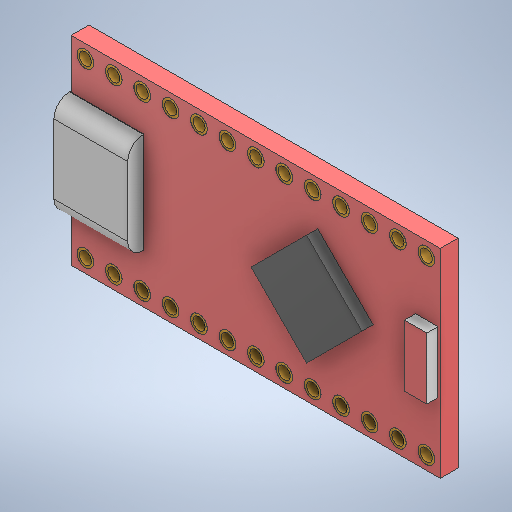
# Autodesk Inventor part: nrf52840
Saved by Autodesk Inventor 2025.2 (Build 292293000, 293)
## iProperties
Created: 2025-04-17
Part Number: nrf52840
Material: Generic
Document SubType Name: Modeling
Designer: Andreas
Density: 1 g/cm^3
Appearance: Default
Author: Andreas
Autodesk Inventor part; units mm, degrees
ref_plane "YZ Plane" through (0, 0, 0) normal (1, 0, 0) x (0, 1, 0)
ref_plane "XZ Plane" through (0, 0, 0) normal (0, 1, 0) x (-1, 0, 0)
ref_plane "XY Plane" through (0, 0, 0) normal (0, 0, 1) x (1, 0, 0)
sketch "Block1" plane through (0, 0, 0) normal (0, 0, 1) x (1, 0, 0)
  line L0 (0.0387, 6.6847) -> (0.0387, 12.8847)
  line L1 (0.2387, 6.6847) -> (0.2387, 12.8847)
  line L2 (1.1887, 12.9847) -> (1.1887, 6.5847)
  line L3 (1.8887, 6.5847) -> (1.8887, 12.9847)
  line L4 (2.8387, 12.8847) -> (2.8387, 6.6847)
  line L5 (3.0387, 12.8847) -> (3.0387, 6.6847)
  arc A0 (1.1887, 6.5847) -> (1.4887, 6.2847) centre (1.4887, 6.5847) ccw
  line L6 (1.4887, 6.2847) -> (1.5887, 6.2847)
  arc A1 (1.5887, 6.2847) -> (1.8887, 6.5847) centre (1.5887, 6.5847) ccw
  arc A2 (1.6387, 5.4847) -> (2.8387, 6.6847) centre (1.6387, 6.6847) ccw
  arc A3 (1.6387, 5.2847) -> (3.0387, 6.6847) centre (1.6387, 6.6847) ccw
  line L7 (1.6387, 5.4847) -> (1.4387, 5.4847)
  line L8 (1.6387, 5.2847) -> (1.4387, 5.2847)
  arc A4 (0.2387, 6.6847) -> (1.4387, 5.4847) centre (1.4387, 6.6847) ccw
  arc A5 (0.0387, 6.6847) -> (1.4387, 5.2847) centre (1.4387, 6.6847) ccw
  line L9 (1.5887, 13.2847) -> (1.4887, 13.2847)
  arc A6 (1.4887, 13.2847) -> (1.1887, 12.9847) centre (1.4887, 12.9847) ccw
  arc A7 (1.8887, 12.9847) -> (1.5887, 13.2847) centre (1.5887, 12.9847) ccw
  arc A8 (2.8387, 12.8847) -> (1.6387, 14.0847) centre (1.6387, 12.8847) ccw
  arc A9 (3.0387, 12.8847) -> (1.6387, 14.2847) centre (1.6387, 12.8847) ccw
  line L10 (1.4387, 14.0847) -> (1.6387, 14.0847)
  arc A10 (1.4387, 14.0847) -> (0.2387, 12.8847) centre (1.4387, 12.8847) ccw
  line L11 (1.4387, 14.2847) -> (1.6387, 14.2847)
  arc A11 (1.4387, 14.2847) -> (0.0387, 12.8847) centre (1.4387, 12.8847) ccw
  point P0 (1.5564, 9.7847)
  point P1 (3.0387, 9.7847)
sketch "Sketch1" plane through (0, 0, 0) normal (0, 0, 1) x (1, 0, 0)
  line L0 (-16.5, -8.9) -> (16.5, -8.9)
  line L1 (16.5, -8.9) -> (16.5, 8.9)
  line L2 (16.5, 8.9) -> (-16.5, 8.9)
  line L3 (-16.5, 8.9) -> (-16.5, -8.9)
  line L4 (-16.5, -8.9) -> (16.5, 8.9) construction
  line L5 (16.5, -8.9) -> (-16.5, 8.9) construction
  point P0 (0, 0)
  dimension "d0" = 33
  dimension "d1" = 17.8
  constraints: 12 end point, 2 midpoint, 2 parallel, 1 horizontal, 1 perpendicular
  measures "d0" distance of L1.end L2.end
  measures "d1" distance of L0.end L1.end
extrude "Extrusion1" add sketch "Sketch1" along normal blind 1.6
sketch "Sketch2" plane through (-16.5, -8.9, 0) normal (-1, 0, 0) x (0, 0, 1)
  line L0 (0, 17.8) -> (0, 0) projected
  line L1 (0.0387, 5.8) -> (0.0387, 12)
  line L2 (0.2387, 5.8) -> (0.2387, 12)
  line L3 (1.1887, 12.1) -> (1.1887, 5.7)
  line L4 (1.8887, 5.7) -> (1.8887, 12.1)
  line L5 (2.8387, 12) -> (2.8387, 5.8)
  line L6 (3.0387, 12) -> (3.0387, 5.8)
  arc A0 (1.1887, 5.7) -> (1.4887, 5.4) centre (1.4887, 5.7) ccw
  line L7 (1.4887, 5.4) -> (1.5887, 5.4)
  arc A1 (1.5887, 5.4) -> (1.8887, 5.7) centre (1.5887, 5.7) ccw
  arc A2 (1.6387, 4.6) -> (2.8387, 5.8) centre (1.6387, 5.8) ccw
  arc A3 (1.6387, 4.4) -> (3.0387, 5.8) centre (1.6387, 5.8) ccw
  line L8 (1.6387, 4.6) -> (1.4387, 4.6)
  line L9 (1.6387, 4.4) -> (1.4387, 4.4)
  arc A4 (0.2387, 5.8) -> (1.4387, 4.6) centre (1.4387, 5.8) ccw
  arc A5 (0.0387, 5.8) -> (1.4387, 4.4) centre (1.4387, 5.8) ccw
  line L10 (1.5887, 12.4) -> (1.4887, 12.4)
  arc A6 (1.4887, 12.4) -> (1.1887, 12.1) centre (1.4887, 12.1) ccw
  arc A7 (1.8887, 12.1) -> (1.5887, 12.4) centre (1.5887, 12.1) ccw
  arc A8 (2.8387, 12) -> (1.6387, 13.2) centre (1.6387, 12) ccw
  arc A9 (3.0387, 12) -> (1.6387, 13.4) centre (1.6387, 12) ccw
  line L11 (1.4387, 13.2) -> (1.6387, 13.2)
  arc A10 (1.4387, 13.2) -> (0.2387, 12) centre (1.4387, 12) ccw
  line L12 (1.4387, 13.4) -> (1.6387, 13.4)
  arc A11 (1.4387, 13.4) -> (0.0387, 12) centre (1.4387, 12) ccw
  point P0 (0, 8.9)
  point P1 (0.0387, 8.9)
  point P2 (0, 8.9)
  constraints: 1 horizontal alignment, 1 midpoint, 1 other
extrude "Extrusion2" add sketch "Sketch2" along normal blind 0.1 and the other way blind 6.5 contours L1 A11 L12 A9 L6 A3 L9 A5 | L2 A10 L11 A8 L5 A2 L8 A4 | A6 L10 A7 L4 A1 L7 A0 L3
extrude "Extrusion3" cut sketch "Sketch2" along normal mid plane 6 contours L2 A10 L11 A8 L5 A2 L8 A4
sketch "Sketch3" plane through (0, 0, 1.6) normal (0, 0, 1) x (1, 0, 0)
  line L0 (0.6005, 0) -> (5.5503, 4.9497)
  line L1 (5.5503, 4.9497) -> (10.5, 0)
  line L2 (10.5, 0) -> (5.5503, -4.9497)
  line L3 (5.5503, -4.9497) -> (0.6005, 0)
  line L4 (0.6005, 0) -> (10.5, 0) construction
  line L5 (5.5503, 4.9497) -> (5.5503, -4.9497) construction
  line L6 (16.5, -8.9) -> (16.5, 8.9) projected
  line L7 (14.3, 2.75) -> (16.3, 2.75)
  line L8 (16.3, 2.75) -> (16.3, -2.75)
  line L9 (16.3, -2.75) -> (14.3, -2.75)
  line L10 (14.3, -2.75) -> (14.3, 2.75)
  point P0 (0, 0)
  point P1 (5.5503, 0)
  point P2 (5.5503, 0)
  point P3 (14.3, 0)
  dimension "d8" = 7
  dimension "d9" = 6
  dimension "d10" = 5.5
  dimension "d11" = 2
  dimension "d12" = 0.2
  constraints: 20 end point, 4 midpoint, 4 parallel, 3 perpendicular, 2 horizontal, 2 horizontal alignment
  measures "d8" distance of L0.end L1.end
  measures "d9" distance from line of L6 L1.end
  measures "d10" distance of L7.end L8.end
  measures "d11" distance of L8.end L9.end
  measures "d12" distance between parallel lines of L6 L8
extrude "Extrusion4" add sketch "Sketch3" along normal blind 1
sketch "Sketch4" plane through (0, 0, 1.6) normal (0, 0, 1) x (1, 0, 0)
  line L0 (-16.5, -4.5) -> (-16.5, -8.9) projected
  line L1 (-10, 3.1) -> (-10, -3.1) projected
  point P0 (0, 0)
  point P1 (-15.23, -7.71)
  point P2 (-10, 0)
  dimension "d22" = 1.27
  dimension "d23" = 7.71
  constraints: 1 midpoint
  measures "d22" distance from line of L0 point (-15.23, -7.71)
  measures "d23" vertical distance of point (-10, 0) point (-15.23, -7.71)
hole "Hole1" at (-15.23, -7.71, 1.6) direction (0, 0, -1) diameter 1.1 end through all counterbore diameter 1.5 counterbore depth 0.01
sketch "Sketch5" plane through (0, 0, 0) normal (0, 0, -1) x (-1, 0, 0)
  circle A0 centre (15.23, -7.71) radius 0.75 projected
  point P0 (0, 0)
extrude "Extrusion5" cut sketch "Sketch5" against normal blind 0.01
pattern_linear "Rectangular Pattern1" count 13 spacing 2.54 along (1, 0, 0) count 2 spacing 15.42 along (0, 1, 0) of "Hole1", "Extrusion5"
body "Solid1"
